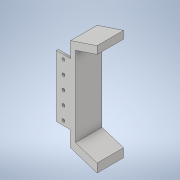
# Autodesk Inventor part: Pala
Saved by Autodesk Inventor 2020 (Build 240168000, 168)
## iProperties
Created: 2019-04-01
Part Number: Pala
Material: Genérico
Document SubType Name: Modeling
Designer: Marcelo
Density: 1 g/cm^3
Appearance: Valor por defecto
Author: Marcelo
Autodesk Inventor part; units mm, degrees
ref_plane "YZ Plane" through (0, 0, 0) normal (1, 0, 0) x (0, 1, 0)
ref_plane "XZ Plane" through (0, 0, 0) normal (0, 1, 0) x (-1, 0, 0)
ref_plane "XY Plane" through (0, 0, 0) normal (0, 0, 1) x (1, 0, 0)
sketch "Boceto1" plane through (0, 0, 0) normal (0, 0, 1) x (1, 0, 0)
  line L0 (-8, 35) -> (8, 35)
  line L1 (8, 35) -> (8, -35)
  line L2 (8, -35) -> (-8, -35)
  line L3 (-8, -35) -> (-8, 35)
  line L4 (-8, 35) -> (8, -35) construction
  line L5 (8, 35) -> (-8, -35) construction
  point P0 (0, 0)
  dimension "d0" = 16
  dimension "d1" = 70
  constraints: 12 end point, 2 midpoint, 2 parallel, 1 horizontal, 1 perpendicular
  measures "d0" distance of L1.end L2.end
  measures "d1" distance of L0.end L1.end
extrude "Extrusión1" add sketch "Boceto1" along normal blind 2
sketch "Boceto2" plane through (0, 0, 2) normal (0, 0, 1) x (1, 0, 0)
  line L0 (38, -62.5) -> (8, -62.5)
  line L1 (8, -62.5) -> (8, 62.5)
  line L2 (8, 62.5) -> (38, 62.5)
  line L3 (38, 62.5) -> (38, -62.5)
  line L4 (38, -62.5) -> (8, 62.5) construction
  line L5 (8, -62.5) -> (38, 62.5) construction
  point P0 (0, 0)
  point P1 (23, 0)
  dimension "d4" = 30
  dimension "d5" = 125
  constraints: 12 end point, 2 midpoint, 2 parallel, 1 horizontal, 1 perpendicular
  measures "d4" distance of L1.end L2.end
  measures "d5" distance of L0.end L1.end
extrude "Extrusión2" add sketch "Boceto2" against normal blind 30
sketch "Boceto3" plane through (0, 0, 2) normal (0, 0, 1) x (1, 0, 0)
  line L0 (38, 62.5) -> (38, -62.5) projected
  line L1 (13.5714, -44.7856) -> (13.5714, 45.755)
  line L2 (38, 45.755) -> (38, -44.7856)
  line L3 (13.5714, -44.7856) -> (38, -52.7345)
  line L4 (38, -52.7345) -> (38, -44.7856)
  line L5 (13.5714, 45.755) -> (38, 53.8978)
  line L6 (38, 45.755) -> (38, 53.8978)
  line L7 (8, -62.5) -> (8, -35) projected
  line L8 (38, -62.5) -> (8, -62.5) projected
  line L9 (8, -62.5) -> (38, -62.5)
  line L10 (38, -62.5) -> (8, -52.7345)
  line L11 (8, -52.7345) -> (8, -62.5)
  line L12 (8, -62.5) -> (8, 62.5) projected
  line L13 (8, 62.5) -> (38, 62.5)
  line L14 (38, 62.5) -> (8, 52.5)
  line L15 (8, 62.5) -> (38, 62.5) projected
  line L16 (8, 52.5) -> (8, 62.5)
  point P0 (0, 0)
  constraints: 24 end point, 5 point on line, 3 collinear, 3 perpendicular, 1 parallel
extrude "Extrusión3" cut sketch "Boceto3" against normal through all contours L14 L12 L13 | L0 L3 L1 L5 | L10 L8 L7
sketch "Boceto4" plane through (0, 0, 0) normal (0, 0, -1) x (-1, 0, 0)
  point P0 (0, 0)
  point P1 (0, 0)
  point P2 (0, 15)
  point P3 (0, 30)
  point P4 (0, -15)
  point P5 (0, -30)
  constraints: 1 coincident
hole "Agujero1" at (0, 0, 0) at (0, 15, 0) at (0, 30, 0) at (0, -15, 0) at (0, -30, 0) direction (0, 0, 1) diameter 3.175 end through all
